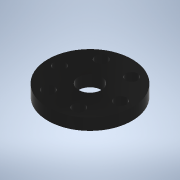
# Autodesk Inventor part: FlywheelSpacer
Saved by Autodesk Inventor 2021 (Build 250183000, 183)
## iProperties
Created: 2021-05-22
Part Number: FlywheelSpacer
Material: PC/ABS Plastic
Document SubType Name: Modeling
Designer: sami8
Density: 0.357273 g/cm^3
Appearance: Smooth - Black
Author: sami8
Autodesk Inventor part; units mm, degrees
ref_plane "YZ Plane" through (0, 0, 0) normal (1, 0, 0) x (0, 1, 0)
ref_plane "XZ Plane" through (0, 0, 0) normal (0, 1, 0) x (-1, 0, 0)
ref_plane "XY Plane" through (0, 0, 0) normal (0, 0, 1) x (1, 0, 0)
sketch "Sketch1" plane through (0, 0, 0) normal (0, 1, 0) x (-1, 0, 0)
  circle A0 centre (0, 0) radius 11
  circle A1 centre (0, 0) radius 8 construction
  circle A2 centre (8, 0) radius 1.55
  line L0 (0, 0) -> (8, 0) construction
  circle A3 centre (4, 6.9282) radius 1.55
  circle A4 centre (-4, 6.9282) radius 1.55
  circle A5 centre (-8, 0) radius 1.55
  circle A6 centre (-4, -6.9282) radius 1.55
  circle A7 centre (4, -6.9282) radius 1.55
  circle A8 centre (0, 0) radius 3
  dimension "d1" = 16
  dimension "d0" = 22
  dimension "d2" = 3.1
  dimension "d5" = 360
  dimension "d9" = 6
  constraints: 8 centre point, 3 coincident, 2 end point, 1 horizontal, 1 horizontal alignment, 15 other
  measures "d0" diameter of A0
  measures "d2" diameter of A2
  measures "d9" diameter of A8
extrude "Extrusion1" add sketch "Sketch1" along normal blind 3
body "Solid1"
